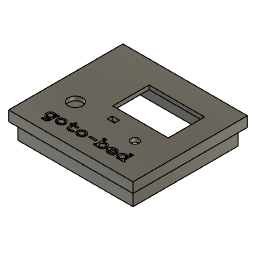
goto-bed (Autodesk Fusion 360 design; units mm, degrees)
Autodesk Fusion 360 part; units mm, degrees
sketch "top" plane through (0, 0, 0) normal (0, 0, 1) x (1, 0, 0)
  line L0 (28.55, -26.05) -> (-28.55, -26.05)
  line L1 (-28.55, -26.05) -> (-28.55, 26.05)
  line L2 (-28.55, 26.05) -> (28.55, 26.05)
  line L3 (28.55, 26.05) -> (28.55, -26.05)
  line L4 (28.55, -26.05) -> (-28.55, 26.05) construction
  line L5 (-28.55, -26.05) -> (28.55, 26.05) construction
  line L6 (30.85, -28.35) -> (-30.85, -28.35)
  line L7 (-30.85, -28.35) -> (-30.85, 28.35)
  line L8 (-30.85, 28.35) -> (30.85, 28.35)
  line L9 (30.85, 28.35) -> (30.85, -28.35)
  line L10 (-6.75, 17.2) -> (20.75, 17.2)
  line L11 (20.75, 17.2) -> (20.75, -0.8)
  line L12 (20.75, -0.8) -> (-6.75, -0.8)
  line L13 (-6.75, -0.8) -> (-6.75, 17.2)
  line L14 (-2.5, -5.3) -> (1, -5.3)
  line L15 (1, -5.3) -> (1, -7.7)
  line L16 (1, -7.7) -> (-2.5, -7.7)
  line L17 (-2.5, -7.7) -> (-2.5, -5.3)
  circle A0 centre (13.75, -10.3) radius 2
  circle A1 centre (-17.75, -8.3) radius 3.5
  line L18 (26.25, -23.75) -> (-26.25, -23.75)
  line L19 (-26.25, -23.75) -> (-26.25, 23.75)
  line L20 (-26.25, 23.75) -> (26.25, 23.75)
  line L21 (26.25, 23.75) -> (26.25, -23.75)
  line L22 (0, 28.35) -> (0, -28.35) construction
  line L23 (-20.6534, -23.35) -> (20.6534, -23.35) construction
  line L24 (20.6534, -23.35) -> (20.6534, -15.8454) construction
  line L25 (20.6534, -15.8454) -> (-20.6534, -15.8454) construction
  line L26 (-20.6534, -15.8454) -> (-20.6534, -23.35) construction
  dimension "d1" = 57.1
  dimension "d2" = 52.1
  dimension "d3" = -2.3
  dimension "d4" = 27.5
  dimension "d5" = 18
  dimension "d10" = 3.5
  dimension "d11" = 2.4
  dimension "d12" = 4.5
  dimension "d13" = 4.25
  dimension "d14" = 4
  dimension "d15" = 7
  dimension "d16" = 25.25
  dimension "d21" = 7.5
  dimension "d22" = 10.75
  dimension "d60" = 2.3
  dimension "d185" = 5.5
  dimension "d186" = 7.5
  dimension "d187" = 4
  text T0 "goto-bed" font "Courier New" height 5 bold align centre middle in box 41.3068 x 7.5046 at (-20.6534, -23.35) x (1, 0) y (0, 1) spacing 1 kerned
  constraint horizontal L0
  constraint perpendicular L0 L1
  constraint parallel L0 L2
  constraint parallel L1 L3
  constraint coincident L4 origin
  constraint coincident L5 origin
  constraint horizontal L10
  constraint vertical L11
  constraint horizontal L12
  constraint vertical L13
  constraint horizontal L14
  constraint vertical L15
  constraint horizontal L16
  constraint vertical L17
  constraint midpoint L8 L22.start
  constraint midpoint L6 L22.end
  constraint perpendicular L22 L25
  constraint coincident L22
  measures "d1" distance of L1.end L2.end
  measures "d2" distance of L0.end L1.end
  measures "d4" distance of L10.start L10.end
  measures "d5" distance of L10.start L12.end
  measures "d10" distance of L14.start L14.end
  measures "d11" distance of L14.start L16.end
  measures "d12" distance of L12 L14
  measures "d13" distance of L12.end L17
  measures "d14" diameter of A0
  measures "d15" diameter of A1
  measures "d16" distance of L0 L12
  measures "d21" distance of L12 A0
  measures "d22" distance of L15 A0
  measures "d185" distance of L11 L21
  measures "d186" distance of L13 A1
  measures "d187" distance of L12 A1
extrude "Extrude2" add sketch "top" against normal blind 2 contours L0 L1 L2 L3 | L6 L7 L8 L9 | L18 L19 L20 L21 makes body 1
extrude "Extrude3" add sketch "top" against normal blind 5 contours L6 L7 L8 L9 bodies 1
extrude "Extrude8" add sketch "top" against normal blind 13 contours L0 L1 L2 L3 bodies 1
sketch "bottom" plane through (0, 0, -5) normal (0, 0, -1) x (1, 0, 0)
  line L0 (26.35, -22.5) -> (-26.35, -22.5)
  line L1 (-26.35, -22.5) -> (-26.35, 22.5)
  line L2 (-26.35, 22.5) -> (26.35, 22.5)
  line L3 (28.65, 24.8) -> (-28.65, 24.8)
  circle A0 centre (0, 0) radius 5
  line L4 (28.55, -26.05) -> (-28.55, -26.05)
  line L5 (-28.55, -26.05) -> (-28.55, 26.05)
  line L6 (-28.55, 26.05) -> (28.55, 26.05)
  line L7 (28.55, 26.05) -> (28.55, -26.05)
  line L8 (-30.85, -28.35) -> (30.85, -28.35)
  line L9 (30.85, -28.35) -> (30.85, 28.35)
  line L10 (30.85, 28.35) -> (-30.85, 28.35)
  line L11 (-30.85, 28.35) -> (-30.85, -28.35)
  line L12 (0, 0) -> (5, 0) construction
  line L13 (5, 0) -> (7.5, 0) construction
  line L14 (0, -2) -> (7.5, -2)
  arc A1 (7.5, -2) -> (7.5, 2) centre (7.5, 0) ccw
  line L15 (7.5, 2) -> (0, 2)
  arc A2 (0, 2) -> (0, -2) centre (0, 0) ccw
  line L16 (0, 0) -> (7.5, 0) construction
  dimension "d67" = 10
  dimension "d131" = 2.5
  dimension "d132" = 2
  constraint coincident A0.centre L12.start
  constraint horizontal L12
  constraint coincident A0 L12.end
  constraint parallel L12 L13
  constraint tangent L14 A1
  constraint tangent A1 L15
  constraint parallel L14 L15
  constraint tangent L15 A2
  constraint tangent L14 A2
  constraint coincident L13.end A1.centre
  constraint parallel L13 L16
  measures "d67" diameter of A0
  measures "d131" distance of L12.end L13.end
  measures "d132" radius of A1
extrude "Extrude9" add sketch "bottom" along normal blind 32 from surface at 0.25 separate body contours L8 L9 L10 L11 makes body 2
extrude "Extrude10" add sketch "bottom" along normal blind 2.5 from surface at 29.75 contours L3 L4 L5 L7 | L3 L5 L6 L7 bodies 2
sketch "bottom_backplate" plane through (0, 0, -34.75) normal (0, 0, 1) x (-1, 0, 0)
  line L0 (-4.5826, -2) -> (-7.5, -2)
  arc A0 (-7.5, 2) -> (-7.5, -2) centre (-7.5, 0) ccw
  line L1 (-7.5, 2) -> (-4.5826, 2)
  line L2 (-28.55, 26.05) -> (-28.55, -26.05)
  line L3 (-28.55, -26.05) -> (28.55, -26.05)
  line L4 (28.55, 26.05) -> (-28.55, 26.05)
  line L5 (28.55, -26.05) -> (-28.55, -26.05)
  line L6 (-28.55, -26.05) -> (-28.55, 26.05)
  line L7 (-28.55, 26.05) -> (28.55, 26.05)
  line L8 (28.55, 26.05) -> (28.55, -26.05)
  line L9 (-4.5826, -2) -> (-4.5826, 2)
  line L10 (-4.5826, -2) -> (-7.5, -2)
  line L11 (-4.5826, 2) -> (-7.5, 2)
  arc A1 (-7.5, 2) -> (-7.5, -2) centre (-7.5, 0) ccw
  line L12 (28.55, -26.05) -> (28.55, 26.05)
  dimension "d137" = 2
  constraint horizontal L5
  constraint vertical L6
  constraint horizontal L7
  constraint vertical L8
  constraint coincident L2.start L4.end
  constraint coincident L3.end L5.start
  constraint coincident L0.start L9.start
  constraint coincident L1.end L9.end
  constraint coincident L0.end A0.end
  constraint coincident A0.start L1.start
  measures "d137" radius of A1
extrude "Extrude11" add sketch "bottom_backplate" along normal blind 3 bodies 2
sketch "right" plane through (30.85, 0, 0) normal (1, 0, 0) x (0, 1, 0)
  line L0 (28.35, -5.25) -> (-28.35, -5.25)
  line L1 (-28.35, -5.25) -> (-28.35, -37.25)
  line L2 (-28.35, -37.25) -> (28.35, -37.25)
  line L3 (28.35, -37.25) -> (28.35, -5.25)
  line L4 (3.9119, -24.15) -> (-3.8381, -24.15)
  line L5 (-3.8381, -24.15) -> (-3.8381, -26.95)
  line L6 (-3.8381, -26.95) -> (3.9119, -26.95)
  line L7 (3.9119, -26.95) -> (3.9119, -24.15)
  line L8 (3.9119, -24.15) -> (-3.8381, -26.95) construction
  line L9 (-3.8381, -24.15) -> (3.9119, -26.95) construction
  line L10 (26.05, -5) -> (-26.05, -5)
  line L11 (-26.05, -5) -> (-26.05, -13)
  line L12 (-26.05, -13) -> (26.05, -13)
  line L13 (26.05, -13) -> (26.05, -5)
  line L14 (28.35, 0) -> (-28.35, 0)
  line L15 (-28.35, 0) -> (-28.35, -5)
  line L16 (-28.35, -5) -> (28.35, -5)
  line L17 (28.35, -5) -> (28.35, 0)
  line L18 (17.2, 0) -> (17.2, -2)
  line L19 (17.2, -2) -> (-0.8, -2)
  line L20 (-0.8, -2) -> (-0.8, 0)
  line L21 (-2, -34.75) -> (2, -34.75)
  line L22 (2, -34.75) -> (2, -31.75)
  line L23 (2, -31.75) -> (-2, -31.75)
  line L24 (-2, -31.75) -> (-2, -34.75)
  line L25 (-0.8, 0) -> (17.2, 0)
  point P0 (0.0369, -25.55)
  dimension "d140" = 7.75
  dimension "d141" = 2.8
  dimension "d145" = 24.15
  dimension "d146" = 0.8
  constraint horizontal L4
  constraint perpendicular L4 L5
  constraint parallel L4 L6
  constraint parallel L5 L7
  constraint coincident L8 P0
  constraint coincident L9 P0
  measures "d140" distance of L5.end L6.end
  measures "d141" distance of L4.end L5.end
  measures "d145" distance of L4 L14
extrude "Extrude12" cut sketch "right" against normal blind 3 contours L4 L5 L6 L7 bodies 2
extrude "Extrude16" cut sketch "top" against normal blind 1.5 text T0 bodies 1
hidden bodies 2
named bodies: "top", "bottom"
